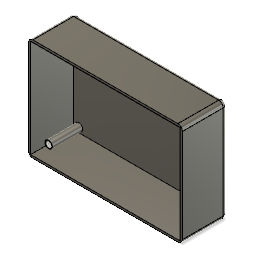
arduino_body v1 (Autodesk Fusion 360 design; units mm, degrees)
Autodesk Fusion 360 part; units mm, degrees
note: some values were not read from the file. Set by a fixed rule: which face or edge a step refers to.
sketch "Sketch1" plane through (0, 0, 0) normal (0, 0, 1) x (1, 0, 0)
  line L0 (-64.77, -43.18) -> (64.77, -43.18)
  line L1 (64.77, -43.18) -> (64.77, 43.18)
  line L2 (64.77, 43.18) -> (-64.77, 43.18)
  line L3 (-64.77, 43.18) -> (-64.77, -43.18)
  line L4 (-64.77, -43.18) -> (64.77, 43.18) construction
  line L5 (64.77, -43.18) -> (-64.77, 43.18) construction
  dimension "d1" = 129.54
  dimension "d2" = 86.36
extrude "Extrude1" add sketch "Sketch1" along normal blind 38.1
shell "Shell1" thickness 2 removed faces 1 at (-21.59, 14.3933, 38.1)
fillet "Fillet1" radius 3.81 4 edges at (0, 43.18, 0) (64.77, 0, 0) (-64.77, 0, 0) (0, -43.18, 0)
fillet "Fillet2" radius 3.81 6 edges at (-63.6541, 42.0641, 1.1159) (-64.77, 43.18, 20.955) (63.6541, 42.0641, 1.1159) (64.77, 43.18, 20.955) (-63.6541, -42.0641, 1.1159) (-64.77, -43.18, 20.955)
fillet "Fillet3" radius 3.81 2 edges at (63.6541, -42.0641, 1.1159) (64.77, -43.18, 20.955)
sketch "Sketch2" plane through (0, 0, 2) normal (0, 0, 1) x (1, 0, 0)
  line L0 (-62.77, 41.18) -> (-62.77, -41.18)
  line L1 (-62.77, -41.18) -> (62.77, -41.18)
  line L2 (62.77, -41.18) -> (62.77, 41.18)
  line L3 (62.77, 41.18) -> (-62.77, 41.18)
  circle A0 centre (-58.6814, 37.2444) radius 3.175
  circle A1 centre (59.0295, 37.8335) radius 3.175
  circle A2 centre (58.8989, -37.3972) radius 3.175
  circle A3 centre (-58.3118, -36.9906) radius 3.175
  dimension "d9" = 6.35
  dimension "d10" = 6.35
  dimension "d12" = 6.35
  dimension "d13" = 6.35
  measures "d9" diameter of A0
  measures "d10" diameter of A1
  measures "d12" diameter of A2
  measures "d13" diameter of A3
extrude "Extrude2" add sketch "Sketch2" along normal blind 25.4 contours A0 | A1 | A2 | A3
shell "Shell2" thickness 0.1 removed faces 4 at (58.3696, 37.0061, 27.4) at (-59.4995, 38.0718, 27.4) at (-59.1298, -36.1632, 27.4) at (58.0808, -36.5698, 27.4)
thread "Thread1" "ANSI Unified Screw Threads 0.25 1/4-20 UNC 3B" major diameter 6.35 minor diameter 5.1156 pitch 1.27 angle 60 resizes the face on face at (62.1006, 37.9868, 18.9) on face at (-55.6103, 37.3976, 18.9) on face at (-55.2406, -36.8373, 18.9) on face at (61.97, -37.244, 18.9)
